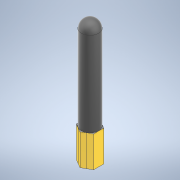
# Autodesk Inventor part: antena
Saved by Autodesk Inventor 2020 (Build 240168000, 168)
## iProperties
Created: 2021-10-19
Part Number: antena
Material: Genérico
Document SubType Name: Modeling
Designer: DANIEL
Density: 1 g/cm^3
Appearance: Valor por defecto
Author: DANIEL
Autodesk Inventor part; units mm, degrees
ref_plane "YZ Plane" through (0, 0, 0) normal (1, 0, 0) x (0, 1, 0)
sketch "Boceto1" plane through (0, 0, 0) normal (0, 1, 0) x (-1, 0, 0)
  circle A0 centre (0, 0) radius 4.5
  dimension "d0" = 9
  constraints: 1 centre point, 1 coincident
  measures "d0" diameter of A0
extrude "Extrusión1" add sketch "Boceto1" along normal blind 64.47
fillet "Empalme1" radius 4.5 1 edges at (4.5, 64.47, 0)
sketch "Boceto2" plane through (0, 0, 0) normal (0, -1, 0) x (1, 0, 0)
  circle A0 centre (0, 0) radius 4.5 projected
  circle A1 centre (0, 0) radius 4.5 projected
  line L0 (3.8723, -2.2357) -> (3.8971, -2.25)
  line L1 (0, 0) -> (5.1962, 0) construction
  line L2 (4.5, -2.5981) -> (4.5, 2.5981)
  line L3 (0, 0) -> (5.1962, 0) construction
  line L4 (4.5, 2.5981) -> (0, 5.1958)
  line L5 (0, 5.1958) -> (-4.5, 2.5981)
  line L6 (-4.5, 2.5981) -> (-4.5409, -2.5978)
  line L7 (-4.5409, -2.5978) -> (-0.0409, -5.1955)
  line L8 (-0.0409, -5.1955) -> (4.5, -2.5981)
  dimension "d9" = 30
  dimension "d11" = 5.196
  dimension "d12" = 5.196
  dimension "d13" = 5.196
  dimension "d14" = 5.196
  constraints: 18 end point, 2 horizontal, 1 parallel, 2 other
  measures "d9" angle of L0 L1
  measures "d11" distance of L2.end L4.end
  measures "d12" distance of L4.end L5.end
  measures "d13" distance of L5.end L6.end
  measures "d14" distance of L6.end L7.end
extrude "Extrusión2" add sketch "Boceto2" against normal blind 16.1175 contours A0 L8 | A0 L2 L8 | A0 L4 L2 | A0 L5 L4 | L8 L7 L6 L5 A0 picked at (-2.0247, -0.1583)
ref_plane "Plano de trabajo1" through (-2.2861, 0, 1.3081) normal (-0.5, 0, -0.8661) x (-0.8661, 0, 0.5)
ref_plane "Plano de trabajo2" through (4.5, 0, -2.5981) normal (0.5, 0, 0.866) x (0, 1, 0)
